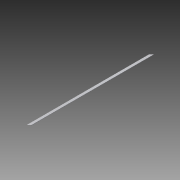
# Autodesk Inventor part: rail aligner
Saved by Autodesk Inventor 2015 SP1 (Build 190203100, 203)
## iProperties
Created: 2015-01-15
Part Number: rail aligner
Material: Nylon, molybdenum disulphide
Document SubType Name: Modeling
Designer: Jarod
Density: 1.13 g/cm^3
Appearance: Nylon 6
Author: Jarod
Autodesk Inventor part; units mm, degrees
ref_plane "YZ Plane" through (0, 0, 0) normal (1, 0, 0) x (0, 1, 0)
ref_plane "XZ Plane" through (0, 0, 0) normal (0, 1, 0) x (-1, 0, 0)
ref_plane "XY Plane" through (0, 0, 0) normal (0, 0, 1) x (1, 0, 0)
sketch "Sketch1" plane through (0, 0, 0) normal (0, 0, 1) x (1, 0, 0)
  line L0 (0, 0) -> (25.4, 0)
  line L1 (25.4, 0) -> (25.4, 3.175)
  line L2 (25.4, 3.175) -> (0, 3.175)
  line L3 (0, 3.175) -> (0, 0)
  dimension "d0" = 25.4
  dimension "d1" = 3.175
  constraints: 8 end point, 2 parallel, 1 horizontal, 1 perpendicular
  measures "d0" distance of L2.end L1.end
  measures "d1" distance of L1.end L0.end
extrude "Extrusion1" add sketch "Sketch1" along normal blind 1689.1
sketch "Sketch2" plane through (0, 3.175, 1689.1) normal (0, 1, 0) x (1, 0, 0)
  line L0 (25.4, 1689.1) -> (0, 1689.1) projected
  line L1 (0, 1689.1) -> (0, 0) projected
  line L2 (25.4, 0) -> (0, 0) projected
  line L3 (25.4, 1689.1) -> (25.4, 0) projected
  point P0 (12.7, 1663.7)
  point P1 (12.7, 12.7)
  dimension "d4" = 12.7
  dimension "d5" = 12.7
  dimension "d6" = 12.7
  dimension "d7" = 25.4
  measures "d4" distance from line of L1 point (12.7, 12.7)
  measures "d5" distance from line of L2 point (12.7, 12.7)
  measures "d6" distance from line of L1 point (12.7, 1663.7)
  measures "d7" distance from line of L0 point (12.7, 1663.7)
hole "Hole1" at (12.7, 3.175, 25.4) at (12.7, 3.175, 1676.4) direction (0, -1, 0) diameter 6.35 end through all
body "Solid1"
